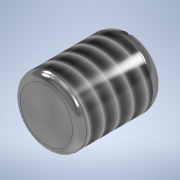
# Autodesk Inventor part: Rans10 punta plana
Saved by Autodesk Inventor 2020 (Build 240168000, 168)
## iProperties
Created: 2020-09-17
Part Number: Rans10 punta plana
Material: Steel AISI 1045 450 QT
Document SubType Name: Modeling
Designer: aaron
Density: 7.85 g/cm^3
Appearance: Steel Galvanized
Author: aaron
Autodesk Inventor part; units mm, degrees
ref_plane "YZ Plane" through (0, 0, 0) normal (1, 0, 0) x (0, 1, 0)
ref_plane "XZ Plane" through (0, 0, 0) normal (0, 1, 0) x (-1, 0, 0)
ref_plane "XY Plane" through (0, 0, 0) normal (0, 0, 1) x (1, 0, 0)
sketch "Sketch1" plane through (0, 0, 0) normal (0, 0, 1) x (1, 0, 0)
  circle A0 centre (0, 0) radius 2.413
  dimension "d0" = 4.826
  constraints: 1 centre point, 1 coincident
  measures "d0" diameter of A0
extrude "Extrusion1" add sketch "Sketch1" along normal blind 6.35
thread "Thread1" size "10-24 UNC" class "2A" standard "ANSI Unified Screw Threads" full length
fillet "Fillet1" radius 0.508 1 edges at (-2.413, 0, 6.35)
fillet "Fillet2" radius 1.016 1 edges at (-2.413, 0, 0)
sketch "Sketch2" plane through (0, 0, 0) normal (0, 0, -1) x (-1, 0, 0)
  line L0 (0.2349, -2.54) -> (-0.2349, -2.54)
  line L1 (-0.2349, -2.54) -> (-0.2349, 2.54)
  line L2 (-0.2349, 2.54) -> (0.2349, 2.54)
  line L3 (0.2349, 2.54) -> (0.2349, -2.54)
  line L4 (0.2349, -2.54) -> (-0.2349, 2.54) construction
  line L5 (-0.2349, -2.54) -> (0.2349, 2.54) construction
  point P0 (0, 0)
  dimension "d7" = 5.08
  dimension "d8" = 0.4697
  constraints: 12 end point, 2 midpoint, 2 parallel, 1 horizontal, 1 perpendicular
  measures "d7" distance of L0.end L1.end
  measures "d8" distance of L1.end L2.end
extrude "Extrusion2" cut sketch "Sketch2" against normal blind 0.762
body "Solid1"
